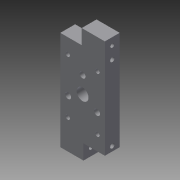
# Autodesk Inventor part: MotorMount
Saved by Autodesk Inventor 2013 (Build 170138000, 138)
## iProperties
Created: 2013-10-23
Part Number: MotorMount
Material: Generic
Document SubType Name: Modeling
Designer: cobrooks
Density: 1 g/cm^3
Author: cobrooks
Autodesk Inventor part; units mm, degrees
ref_plane "YZ Plane" through (0, 0, 0) normal (1, 0, 0) x (0, 1, 0)
ref_plane "XZ Plane" through (0, 0, 0) normal (0, 1, 0) x (-1, 0, 0)
ref_plane "XY Plane" through (0, 0, 0) normal (0, 0, 1) x (1, 0, 0)
sketch "Sketch1" plane through (0, 0, 0) normal (0, 0, 1) x (1, 0, 0)
  line L0 (-19.05, -48.7045) -> (19.05, -48.7045)
  line L1 (19.05, -48.7045) -> (19.05, 48.7045)
  line L2 (19.05, 48.7045) -> (-19.05, 48.7045)
  line L3 (-19.05, 48.7045) -> (-19.05, -48.7045)
  line L4 (-19.05, -48.7045) -> (19.05, 48.7045) construction
  line L5 (19.05, -48.7045) -> (-19.05, 48.7045) construction
  point P0 (0, 0)
  dimension "d0" = 38.1
  dimension "d1" = 97.409
  constraints: 12 end point, 2 midpoint, 2 parallel, 1 horizontal, 1 perpendicular
  measures "d0" distance of L2.end L1.end
  measures "d1" distance of L1.end L0.end
extrude "Extrusion1" add sketch "Sketch1" along normal blind 12.7
sketch "Sketch2" plane through (0, 0, 12.7) normal (0, 0, 1) x (1, 0, 0)
  line L0 (-19.05, 48.7045) -> (-0.762, 48.7045)
  line L1 (-0.762, 48.7045) -> (-0.762, 36.0045)
  line L2 (-0.762, 36.0045) -> (-19.05, 36.0045)
  line L3 (-19.05, 36.0045) -> (-19.05, 48.7045)
  point P0 (0, 0)
  dimension "d4" = 18.288
  dimension "d5" = 12.7
  constraints: 8 end point, 2 parallel, 1 horizontal, 1 perpendicular
  measures "d4" distance of L1.end L2.end
  measures "d5" distance of L0.end L1.end
extrude "Extrusion2" cut sketch "Sketch2" against normal blind 12.7
sketch "Sketch3" plane through (0, 0, 12.7) normal (0, 0, 1) x (1, 0, 0)
  line L0 (19.05, -48.7045) -> (0.762, -48.7045)
  line L1 (0.762, -48.7045) -> (0.762, -36.0045)
  line L2 (0.762, -36.0045) -> (19.05, -36.0045)
  line L3 (19.05, -36.0045) -> (19.05, -48.7045)
  point P0 (0, 0)
  dimension "d8" = 18.288
  dimension "d9" = 12.7
  constraints: 8 end point, 2 parallel, 1 horizontal, 1 perpendicular
  measures "d8" distance of L1.end L2.end
  measures "d9" distance of L0.end L1.end
extrude "Extrusion3" cut sketch "Sketch3" against normal blind 12.7
sketch "Sketch4" plane through (0, 0, 12.7) normal (0, 0, 1) x (1, 0, 0)
  circle A0 centre (0, 0) radius 5.08
  dimension "d12" = 10.16
  constraints: 1 centre point, 1 coincident
  measures "d12" diameter of A0
extrude "Extrusion4" cut sketch "Sketch4" against normal blind 12.7
sketch "Sketch5" plane through (19.05, 48.7045, 12.7) normal (1, 0, 0) x (0, 0, -1)
  line L0 (12.7, -97.409) -> (12.7, 0) projected
  line L1 (12.7, 0) -> (0, 0) projected
  line L2 (0, -84.709) -> (0, 0) projected
  line L3 (0, -12.7) -> (12.7, -12.7) projected
  circle A0 centre (6.35, -6.35) radius 1.5875
  point P0 (12.7, -48.7045)
  dimension "d16" = 3.175
  dimension "d17" = 6.35
  dimension "d18" = 6.35
  dimension "d19" = 6.35
  dimension "d20" = 6.35
  constraints: 1 centre point
  measures "d16" diameter of A0
  measures "d17" distance from line of L0 A0.centre
  measures "d18" distance from line of L2 A0.centre
  measures "d19" distance from line of L3 A0.centre
  measures "d20" distance from line of L1 A0.centre
extrude "Extrusion5" cut sketch "Sketch5" against normal blind 34.29 contours A0
sketch "Sketch9" plane through (-19.05, -48.7045, 0) normal (-1, 0, 0) x (0, 0, 1)
  line L0 (0, 0) -> (12.7, 0) projected
  line L1 (12.7, 84.709) -> (12.7, 0) projected
  line L2 (12.7, 12.709) -> (0, 12.709) projected
  circle A0 centre (6.35, 6.35) radius 1.5875
  line L3 (12.7, 12.7) -> (0, 12.7) projected
  point P0 (0, 48.7045)
  dimension "d34" = 3.175
  dimension "d35" = 6.35
  dimension "d40" = 6.35
  dimension "d41" = 6.35
  constraints: 1 centre point
  measures "d34" diameter of A0
  measures "d35" distance from line of L1 A0.centre
  measures "d40" distance from line of L0 A0.centre
  measures "d41" distance from line of L3 A0.centre
extrude "Extrusion9" cut sketch "Sketch9" against normal blind 20.701
sketch "Sketch10" plane through (0, 0, 12.7) normal (0, 0, 1) x (1, 0, 0)
  circle A0 centre (0, 0) radius 5.08 projected
  line L0 (0.762, -36.0045) -> (19.05, -36.0045) projected
  line L1 (4.0695, 16.6582) -> (16.4611, -4.8048)
  line L2 (12.3917, -11.8533) -> (-12.3917, -11.8533)
  line L3 (-16.4611, -4.8048) -> (-4.0695, 16.6582)
  line L4 (-1.524, 36.0045) -> (-1.524, -36.0045) construction
  arc A1 (-16.4611, -4.8048) -> (-12.3917, -11.8533) centre (-12.3917, -7.1543) ccw
  arc A2 (4.0695, 16.6582) -> (-4.0695, 16.6582) centre (0, 14.3087) ccw
  arc A3 (12.3917, -11.8533) -> (16.4611, -4.8048) centre (12.3917, -7.1543) ccw
  circle A4 centre (-12.3917, -7.1543) radius 2.54
  circle A5 centre (0, 14.3087) radius 2.54
  circle A6 centre (12.3917, -7.1543) radius 2.54
  point P0 (-0.762, 36.0045)
  point P1 (0, 23.7067)
  point P2 (20.5306, -11.8533)
  point P3 (-20.5306, -11.8533)
  dimension "d52" = 35.56
  dimension "d53" = 4.699
  dimension "d54" = 4.699
  dimension "d55" = 5.08
  dimension "d56" = 5.08
  dimension "d57" = 5.08
  constraints: 8 end point, 6 centre point, 6 point on circle, 6 point on line, 6 tangent, 4 coincident, 1 equal radius, 1 parallel, 1 perpendicular, 7 other
  measures "d52" distance from line of point (0, 23.707) L2
  measures "d53" radius of A1
  measures "d54" radius of A2
  measures "d55" diameter of A4
  measures "d56" diameter of A5
  measures "d57" diameter of A6
extrude "Extrusion11" cut sketch "Sketch10" against normal blind 12.7 contours A4 | A5 | A6
sketch "Sketch11" plane through (19.05, 48.7045, 12.7) normal (1, 0, 0) x (0, 0, -1)
  circle A0 centre (6.35, -16.7) radius 1.85 projected
  circle A1 centre (6.35, -80.7) radius 1.85 projected
  point P0 (12.7, -48.7045)
extrude "Extrusion12" cut sketch "Sketch11" against normal blind 38.1
sketch "Sketch12" plane through (0, 0, 12.7) normal (0, 0, 1) x (1, 0, 0)
  line L0 (0.762, -36.0045) -> (19.05, -36.0045) projected
  line L1 (19.05, -36.0045) -> (19.05, 48.7045) projected
  line L2 (-0.762, 36.0045) -> (-19.05, 36.0045) projected
  line L3 (-19.05, 36.0045) -> (-19.05, -48.7045) projected
  circle A0 centre (-12.7, 23.3045) radius 1.8542
  circle A1 centre (12.7, 23.3045) radius 1.8542
  circle A2 centre (12.7, -23.3045) radius 1.8542
  circle A3 centre (-12.7, -23.3045) radius 1.8542
  dimension "d62" = 3.7084
  dimension "d64" = 6.35
  dimension "d65" = 12.7
  dimension "d66" = 3.7084
  dimension "d67" = 12.7
  dimension "d68" = 6.35
  dimension "d69" = 3.7084
  dimension "d70" = 6.35
  dimension "d71" = 12.7
  dimension "d72" = 3.7084
  dimension "d73" = 6.35
  dimension "d74" = 12.7
  constraints: 4 centre point
  measures "d62" diameter of A0
  measures "d64" distance from line of L3 A0.centre
  measures "d65" distance from line of L2 A0.centre
  measures "d66" diameter of A1
  measures "d67" distance from line of A1.centre L2
  measures "d68" distance from line of L1 A1.centre
  measures "d69" diameter of A2
  measures "d70" distance from line of L1 A2.centre
  measures "d71" distance from line of L0 A2.centre
  measures "d72" diameter of A3
  measures "d73" distance from line of L3 A3.centre
  measures "d74" distance from line of A3.centre L0
extrude "Extrusion13" cut sketch "Sketch12" against normal blind 12.7
equation "\"d17\" = d18"
equation "\"d19\" = d20"
equation "\"d40\" = d41"
body "Solid1"
